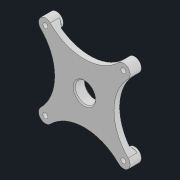
# Autodesk Inventor part: Part1
Saved by Autodesk Inventor 2022 (Build 260153000, 153)
## iProperties
Created: 2021-10-28
Part Number: Part1
Material: 一般
Document SubType Name: Modeling
Designer: Yuta Kage
Density: 1 g/cm^3
Appearance: 既定
Author: Yuta Kage
Autodesk Inventor part; units mm, degrees
ref_plane "YZ Plane" through (0, 0, 0) normal (1, 0, 0) x (0, 1, 0)
ref_plane "XZ Plane" through (0, 0, 0) normal (0, 1, 0) x (-1, 0, 0)
ref_plane "XY Plane" through (0, 0, 0) normal (0, 0, 1) x (1, 0, 0)
sketch "スケッチ1" plane through (0, 0, 0) normal (0, 0, 1) x (1, 0, 0)
  circle A0 centre (0, 0) radius 49 construction
  circle A1 centre (-34.648232, 34.648232) radius 6
  circle A2 centre (-34.648232, -34.648232) radius 6
  circle A3 centre (34.648232, -34.648232) radius 6
  circle A4 centre (34.648232, 34.648232) radius 6
  circle A5 centre (0, 69.296465) radius 43
  circle A6 centre (-69.296465, 0) radius 43
  circle A7 centre (0, -69.296465) radius 43
  circle A8 centre (69.296465, 0) radius 43
  line L0 (-40.648232, -40.648232) -> (40.648232, -40.648232)
  line L1 (40.648232, -40.648232) -> (40.648232, 40.648232)
  line L2 (40.648232, 40.648232) -> (-40.648232, 40.648232)
  line L3 (-40.648232, 40.648232) -> (-40.648232, -40.648232)
  line L4 (-40.648232, -40.648232) -> (40.648232, 40.648232) construction
  line L5 (40.648232, -40.648232) -> (-40.648232, 40.648232) construction
  line L6 (0, 69.296465) -> (-69.296465, 0)
  circle A9 centre (0, 0) radius 13
  point P0 (0, 26.296465)
  point P1 (-26.296465, 0)
  point P2 (0, -26.296465)
  point P3 (26.296465, 0)
  point P4 (38.890873, -30.405592)
  point P5 (38.890873, 30.405592)
  point P6 (30.405592, 38.890873)
  point P7 (-30.405592, 38.890873)
  point P8 (-38.890873, 30.405592)
  point P9 (-38.890873, -30.405592)
  point P10 (-30.405592, -38.890873)
  point P11 (30.405592, -38.890873)
  dimension "d0" = 98
  dimension "d1" = 12
  dimension "d4" = 360
  dimension "d9" = 360
  dimension "d27" = 26
  constraints: 14 end point, 5 centre point, 3 midpoint, 2 coincident, 2 parallel, 2 tangent, 1 horizontal, 1 horizontal alignment, 1 perpendicular, 1 vertical alignment, 39 other
  measures "d1" diameter of A1
  measures "d27" diameter of A9
extrude "押し出し1" add sketch "スケッチ1" along normal blind 5 contours A1 L6 | A1 A5 A4 A8 A3 A7 A2 A6 | L6 A1 | A4 | A2 | A3 | A9
extrude "押し出し4" add sketch "スケッチ1" against normal blind 5 contours A1 L6 | L6 A1 | A4 | A2 | A3
sketch "スケッチ6" plane through (-34.648232, -34.648232, -5) normal (0, 0, -1) x (-1, 0, 0)
  circle A0 centre (-69.296465, 0) radius 6
  circle A1 centre (0, 0) radius 6
  circle A2 centre (0, 69.296465) radius 6
  circle A3 centre (-69.296465, 69.296465) radius 6
  point P0 (-34.648232, 34.648232)
hole "穴1" at (-34.648232, -34.648232, -5) at (34.648232, -34.648232, -5) at (-34.648232, 34.648232, -5) at (34.648232, 34.648232, -5) direction (0, 0, 1) diameter 4.5 end through all clearance for "Flat Head Machine Screw" size "M4" standard "Ansi Metric M Profile"
sketch "スケッチ7" plane through (0, 0, 0) normal (0, 0, -1) x (-1, 0, 0)
  circle A0 centre (0, 0) radius 13
  dimension "d38" = 26
  constraints: 1 centre point, 1 coincident
  measures "d38" diameter of A0
extrude "押し出し6" add sketch "スケッチ7" along normal blind 5
sketch "スケッチ8" plane through (0, 0, -5) normal (0, 0, -1) x (-1, 0, 0)
  circle A0 centre (0, 0) radius 9
  dimension "d41" = 18
  constraints: 1 centre point, 1 coincident
  measures "d41" diameter of A0
extrude "押し出し7" cut sketch "スケッチ8" against normal through all
chamfer "面取り1" distance 1 angle 45 2 edges at (9, 0, 5) (9, 0, -5)
chamfer "面取り2" distance 3 angle 45 7 edges at (-29.105, -36.9443, 0) (-32.3521, -29.105, 0) (30.4056, -30.4056, 0) (-29.105, 36.9443, 0) (-32.3521, 29.105, 0) (30.4056, 30.4056, 0) (13, 0, 0)
